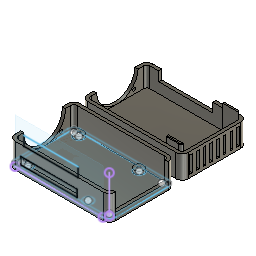
RasPi + Relay Shield (Autodesk Fusion 360 design; units mm, degrees)
Autodesk Fusion 360 part; units mm, degrees
sketch "Sketch1" plane through (0, 0, 0) normal (0, 0, 1) x (1, 0, 0)
  line L0 (-22.9024, 22.7432) -> (61.5976, 22.7432)
  line L1 (64.5976, 19.7432) -> (64.5976, -30.7568)
  line L2 (61.5976, -33.7568) -> (-22.9024, -33.7568)
  line L3 (-25.9024, -30.7568) -> (-25.9024, 19.7432)
  arc A0 (-22.9024, 22.7432) -> (-25.9024, 19.7432) centre (-22.9024, 19.7432) ccw
  arc A1 (-25.9024, -30.7568) -> (-22.9024, -33.7568) centre (-22.9024, -30.7568) ccw
  arc A2 (61.5976, -33.7568) -> (64.5976, -30.7568) centre (61.5976, -30.7568) ccw
  arc A3 (64.5976, 19.7432) -> (61.5976, 22.7432) centre (61.5976, 19.7432) ccw
  circle A4 centre (-17.4024, -30.0068) radius 1.625
  circle A5 centre (40.5976, -30.0068) radius 1.625
  circle A6 centre (40.5976, 18.9932) radius 1.625
  circle A7 centre (-17.4024, 18.9932) radius 1.625
  arc A8 (-22.9024, 25.7432) -> (-28.9024, 19.7432) centre (-22.9024, 19.7432) ccw
  line L4 (-28.9024, -30.7568) -> (-28.9024, 19.7432)
  arc A9 (-28.9024, -30.7568) -> (-22.9024, -36.7568) centre (-22.9024, -30.7568) ccw
  line L5 (61.5976, -36.7568) -> (-22.9024, -36.7568)
  arc A10 (61.5976, -36.7568) -> (67.5976, -30.7568) centre (61.5976, -30.7568) ccw
  line L6 (67.5976, 19.7432) -> (67.5976, -30.7568)
  arc A11 (67.5976, 19.7432) -> (61.5976, 25.7432) centre (61.5976, 19.7432) ccw
  line L7 (-22.9024, 25.7432) -> (61.5976, 25.7432)
  circle A12 centre (-17.4024, 18.9932) radius 4.5
  circle A13 centre (40.5976, 18.9932) radius 4.5
  circle A14 centre (-17.4024, -30.0068) radius 4.5
  circle A15 centre (40.5976, -30.0068) radius 4.5
  line L8 (64.5976, -30.7568) -> (67.5976, -30.7568)
  line L9 (64.5976, 19.7432) -> (67.5976, 19.7432)
  line L10 (-28.9024, 14.4932) -> (-25.9024, 14.4932)
  line L11 (-28.9024, -25.5068) -> (-25.9024, -25.5068)
  point P0 (-25.9024, 22.7432)
  point P1 (64.5976, 22.7432)
  point P2 (-25.9024, -33.7568)
  dimension "d1" = 90.5
  dimension "d2" = 56.5
  dimension "d3" = 3
  dimension "d4" = 3
  dimension "d5" = 3
  dimension "d6" = 3
  dimension "d8" = 3.25
  dimension "d9" = 3.25
  dimension "d10" = 3.25
  dimension "d12" = 58
  dimension "d14" = 3.25
  dimension "d15" = 3.75
  dimension "d18" = 49
  dimension "d20" = 3.75
  dimension "d21" = 58
  dimension "d22" = 3
  dimension "d23" = 49
  dimension "d24" = 9
  dimension "d25" = 9
  dimension "d26" = 9
  dimension "d27" = 9
  dimension "d28" = 40
  dimension "d29" = 11.25
  dimension "d65" = 24
  constraint perpendicular L0 L1
  constraint parallel L0 L2
  constraint parallel L1 L3
  constraint horizontal L0
  constraint coincident P0 L0
  constraint coincident P0 L3
  constraint tangent L0 A0
  constraint tangent L3 A0
  constraint coincident P2 L3
  constraint coincident P2 L2
  constraint tangent L3 A1
  constraint tangent L2 A1
  constraint tangent L2 A2
  constraint tangent L1 A2
  constraint coincident P1 L0
  constraint coincident P1 L1
  constraint tangent L0 A3
  constraint tangent L1 A3
  constraint concentric A7 A12
  constraint concentric A6 A13
  constraint concentric A4 A14
  constraint concentric A5 A15
  constraint perpendicular L1 L8
  constraint perpendicular L6 L9
  constraint coincident L4 L10.start
  constraint coincident L3 L10.end
  constraint perpendicular L3 L10
  constraint coincident L4 L11.start
  constraint coincident L3 L11.end
  constraint perpendicular L3 L11
  measures "d1" distance of P0 P1
  measures "d2" distance of P0 P2
  measures "d3" radius of A0
  measures "d4" radius of A1
  measures "d5" radius of A2
  measures "d6" radius of A3
  measures "d8" diameter of A4
  measures "d9" diameter of A5
  measures "d10" diameter of A6
  measures "d12" horizontal distance of A4.centre A5.centre
  measures "d14" diameter of A7
  measures "d15" distance of L0 A7.centre
  measures "d18" distance of A4.centre A7.centre
  measures "d20" distance of L0 A6.centre
  measures "d21" distance of A6.centre A7.centre
  measures "d22" distance of A0
  measures "d23" distance of A5.centre A6.centre
  measures "d24" diameter of A12
  measures "d25" diameter of A13
  measures "d26" diameter of A14
  measures "d27" diameter of A15
  measures "d28" distance of L10 L11
  measures "d29" distance of L5 L11
  measures "d65" distance of L1 A6.centre
extrude "Extrude1" add sketch "Sketch1" against normal blind 3 makes body 1
extrude "Extrude2" add sketch "Sketch1" along normal blind 3 contours L0 A12 | L0 A12 | L0 A13 | L0 A13 | L2 A14 | L2 A14 | L2 A15 | L2 A15 bodies 1
extrude "Extrude3" add sketch "Sketch1" along normal blind 4 contours L1 L6 L8 L9 bodies 1
extrude "Extrude4" add sketch "Sketch1" along normal blind 40 contours L0 L3 A0 A3 A8 L4 A11 L7 A12 A13 L9 L10 | L0 A12 | L0 A13 | L2 L3 A1 A2 L4 A9 L5 A10 A14 A15 L8 L11 | L2 A14 | L2 A15 picked at (-17.1836, 22.9772) picked at (41.0077, 23.0848) picked at (-16.7645, -33.8643) picked at (41.2355, -33.8643) bodies 1
sketch "Sketch2" plane through (-28.9024, 0, 0) normal (-1, 0, 0) x (0, -1, 0)
  line L0 (25.5068, 0) -> (-14.4932, 0)
  line L1 (-14.4932, 0) -> (-14.4932, 40)
  line L2 (-14.4932, 40) -> (-19.7432, 40)
  line L3 (-19.7432, 40) -> (-19.7432, -3)
  line L4 (-19.7432, -3) -> (30.7568, -3)
  line L5 (30.7568, -3) -> (30.7568, 40)
  line L6 (30.7568, 40) -> (25.5068, 40)
  line L7 (25.5068, 40) -> (25.5068, 0)
  circle A0 centre (5.5068, 20) radius 20
  line L8 (30.7568, 0) -> (-19.7432, 0)
  line L9 (-14.4932, 40) -> (25.5068, 40)
  circle A1 centre (-10.4932, 36) radius 1.45
  circle A2 centre (21.5068, 36) radius 1.45
  circle A3 centre (-10.4932, 4) radius 1.45
  circle A4 centre (21.5068, 4) radius 1.45
  dimension "d38" = 40
  dimension "d39" = 20
  dimension "d40" = 20
  dimension "d41" = 2.9
  dimension "d42" = 4
  dimension "d43" = 4
  dimension "d46" = 32
  dimension "d47" = -32
  constraint coincident L1.end L2.start
  constraint coincident L6.end L7.start
  measures "d38" diameter of A0
  measures "d39" distance of L7 A0.centre
  measures "d40" distance of A0.centre L8
  measures "d41" diameter of A1
  measures "d42" distance of L9 A1.centre
  measures "d43" distance of L1 A1.centre
extrude "Extrude5" add sketch "Sketch2" against normal blind 3 contours L0 L7 A0 L8 | L0 L1 A0 L8 | L7 A0 L9 | L1 A0 L9 bodies 1
extrude "Extrude6" add sketch "Sketch1" along normal blind 3 from surface at 40 contours L0 L3 A0 A3 A8 L4 A11 L7 A12 A13 L9 L10 | L0 L1 L2 L3 A0 A1 A2 A3 A12 A13 A14 A15 | L0 A12 | L0 A12 | L3 L4 L10 L11 | L0 A13 | L0 A13 | L2 L3 A1 A2 L4 A9 L5 A10 A14 A15 L8 L11 | L1 L6 L8 L9 | L2 A14 | L2 A14 | L2 A15 | L2 A15 | A4 | A5 | A6 | A7 bodies 1
sketch "Sketch3" plane through (0, -36.7568, 0) normal (0, -1, 0) x (1, 0, 0)
  line L0 (-22.9024, 43) -> (-22.9024, -3)
  line L1 (-22.9024, -3) -> (61.5976, -3)
  line L2 (61.5976, -3) -> (61.5976, 43)
  line L3 (61.5976, 43) -> (-22.9024, 43)
  line L4 (61.5976, 0) -> (-22.9024, 0)
  line L5 (-17.4024, 11) -> (-17.4024, 4)
  line L6 (-17.4024, 4) -> (36.5976, 4)
  line L7 (36.5976, 4) -> (36.5976, 11)
  line L8 (36.5976, 11) -> (-17.4024, 11)
  line L9 (-14.4024, 21) -> (37.5976, 21)
  line L10 (-14.4024, 21) -> (-14.4024, 30)
  line L11 (37.5976, 21) -> (37.5976, 30)
  line L12 (37.5976, 30) -> (-14.4024, 30)
  line L13 (67.5976, 4) -> (67.5976, 40)
  dimension "d56" = 7
  dimension "d57" = 54
  dimension "d58" = 4
  dimension "d59" = 21
  dimension "d60" = 52
  dimension "d62" = 9
  dimension "d68" = 30
  dimension "d69" = 31
  constraint perpendicular L5 L6
  constraint parallel L5 L7
  constraint parallel L6 L8
  constraint vertical L5
  constraint horizontal L9
  constraint perpendicular L9 L10
  constraint parallel L10 L11
  measures "d56" distance of L5.start L5.end
  measures "d57" distance of L5.start L7.end
  measures "d58" distance of L4 L6
  measures "d59" distance of L4 L9
  measures "d60" distance of L9.start L9.end
  measures "d62" distance of L9.start L10.end
  measures "d68" distance of L11 L13
  measures "d69" distance of L7 L13
extrude "Extrude7" cut sketch "Sketch3" against normal blind 3 contours L5 L6 L7 L8 | L9 L10 L11 L12 bodies 1
ref_plane "WorkPlane1" through (19.3476, -5.5068, 21) normal (0, 0, 1) x (1, 0, 0)
sketch "Sketch4" plane through (0, 0, 40) normal (0, 0, -1) x (1, 0, 0)
  line L0 (64.5976, -19.7432) -> (67.5976, -19.7432)
  line L1 (67.5976, -19.7432) -> (67.5976, 30.7568)
  line L2 (67.5976, 30.7568) -> (64.5976, 30.7568)
  arc A0 (64.5976, 30.7568) -> (61.5976, 33.7568) centre (61.5976, 30.7568) ccw
  line L3 (61.5976, 33.7568) -> (-22.9024, 33.7568)
  arc A1 (-22.9024, 33.7568) -> (-25.9024, 30.7568) centre (-22.9024, 30.7568) ccw
  line L4 (-25.9024, 30.7568) -> (-25.9024, 5.5068)
  line L5 (-25.9024, 5.5068) -> (-25.9024, -19.7432)
  arc A2 (-25.9024, -19.7432) -> (-22.9024, -22.7432) centre (-22.9024, -19.7432) ccw
  line L6 (-22.9024, -22.7432) -> (61.5976, -22.7432)
  arc A3 (61.5976, -22.7432) -> (64.5976, -19.7432) centre (61.5976, -19.7432) ccw
  line L7 (64.5976, 30.7568) -> (64.5976, -19.7432)
  constraint coincident L2.end A0.start
  constraint coincident L0.start A3.end
extrude "Extrude8" add sketch "Sketch4" along normal blind 19 contours L0 L1 L2 L7 bodies 1
sketch "Sketch5" plane through (67.5976, 0, 0) normal (1, 0, 0) x (0, 1, 0)
  line L0 (19.7432, 21) -> (19.7432, 43)
  line L1 (19.7432, 43) -> (-30.7568, 43)
  line L2 (-30.7568, 43) -> (-30.7568, 21)
  line L3 (-30.7568, 21) -> (19.7432, 21)
  line L4 (-29.2586, 40) -> (-29.2586, 24)
  line L5 (-29.2586, 24) -> (-26.7586, 24)
  line L6 (-26.7586, 24) -> (-26.7586, 40)
  line L7 (-26.7586, 40) -> (-29.2586, 40)
  line L8 (-30.7568, 40) -> (-5.5068, 40)
  line L9 (-20.33, 24) -> (-20.33, 40)
  line L10 (-20.33, 40) -> (-22.83, 40)
  line L11 (-22.83, 40) -> (-22.83, 24)
  line L12 (-22.83, 24) -> (-20.33, 24)
  line L13 (-13.9015, 24) -> (-13.9015, 40)
  line L14 (-13.9015, 40) -> (-16.4015, 40)
  line L15 (-16.4015, 40) -> (-16.4015, 24)
  line L16 (-16.4015, 24) -> (-13.9015, 24)
  line L17 (-7.4729, 24) -> (-7.4729, 40)
  line L18 (-7.4729, 40) -> (-9.9729, 40)
  line L19 (-9.9729, 40) -> (-9.9729, 24)
  line L20 (-9.9729, 24) -> (-7.4729, 24)
  line L21 (-1.0443, 24) -> (-1.0443, 40)
  line L22 (-1.0443, 40) -> (-3.5443, 40)
  line L23 (-3.5443, 40) -> (-3.5443, 24)
  line L24 (-3.5443, 24) -> (-1.0443, 24)
  line L25 (5.3842, 24) -> (5.3842, 40)
  line L26 (5.3842, 40) -> (2.8842, 40)
  line L27 (2.8842, 40) -> (2.8842, 24)
  line L28 (2.8842, 24) -> (5.3842, 24)
  line L29 (11.8128, 24) -> (11.8128, 40)
  line L30 (11.8128, 40) -> (9.3128, 40)
  line L31 (9.3128, 40) -> (9.3128, 24)
  line L32 (9.3128, 24) -> (11.8128, 24)
  line L33 (18.2414, 24) -> (18.2414, 40)
  line L34 (18.2414, 40) -> (15.7414, 40)
  line L35 (15.7414, 40) -> (15.7414, 24)
  line L36 (15.7414, 24) -> (18.2414, 24)
  dimension "d73" = 2.5
  dimension "d76" = 45
  dimension "d77" = 0
  constraint perpendicular L4 L5
  constraint parallel L4 L6
  constraint parallel L5 L7
  constraint perpendicular L4 L8
  constraint coincident L4.start L8
  measures "d73" distance of L4.start L6.end
extrude "Extrude9" cut sketch "Sketch5" against normal up to surface (3 mm away) contours L4 L5 L6 L7 L8 | L8 L9 L10 L11 L12 | L8 L13 L14 L15 L16 | L8 L17 L18 L19 L20 | L21 L22 L23 L24 | L25 L26 L27 L28 | L29 L30 L31 L32 | L33 L34 L35 L36 bodies 1
split "Split2" by plane through (19.3476, -5.5068, 21) normal (0, 0, 1) bodies 1 makes body 2 at (33.4309, -15.9234, 43)
move_body "Move1" bodies 2 to x (1, 0, 0) y (0, -1, 0) z (0, 0, -1) at (0, 58.9865, 40)
sketch "Sketch6" plane through (0, 0, 0) normal (0, 0, 1) x (-1, 0, 0)
  line L0 (-64.5976, -39.2432) -> (-64.5976, -40.7451)
  line L1 (-64.5976, -40.7451) -> (-67.5976, -40.7451)
  line L2 (-67.5976, -40.7451) -> (-67.5976, -43.2451)
  line L3 (-67.5976, -43.2451) -> (-64.5976, -43.2451)
  line L4 (-64.5976, -43.2451) -> (-64.5976, -47.1737)
  line L5 (-64.5976, -47.1737) -> (-67.5976, -47.1737)
  line L6 (-67.5976, -47.1737) -> (-67.5976, -49.6737)
  line L7 (-67.5976, -49.6737) -> (-64.5976, -49.6737)
  line L8 (-64.5976, -49.6737) -> (-64.5976, -53.6022)
  line L9 (-64.5976, -53.6022) -> (-67.5976, -53.6022)
  line L10 (-67.5976, -53.6022) -> (-67.5976, -56.1022)
  line L11 (-67.5976, -56.1022) -> (-64.5976, -56.1022)
  line L12 (-64.5976, -56.1022) -> (-64.5976, -60.0308)
  line L13 (-64.5976, -60.0308) -> (-67.5976, -60.0308)
  line L14 (-67.5976, -60.0308) -> (-67.5976, -62.5308)
  line L15 (-67.5976, -62.5308) -> (-64.5976, -62.5308)
  line L16 (-64.5976, -62.5308) -> (-64.5976, -66.4594)
  line L17 (-64.5976, -66.4594) -> (-67.5976, -66.4594)
  line L18 (-67.5976, -66.4594) -> (-67.5976, -68.9594)
  line L19 (-67.5976, -68.9594) -> (-64.5976, -68.9594)
  line L20 (-64.5976, -68.9594) -> (-64.5976, -72.888)
  line L21 (-64.5976, -72.888) -> (-67.5976, -72.888)
  line L22 (-67.5976, -72.888) -> (-67.5976, -75.388)
  line L23 (-67.5976, -75.388) -> (-64.5976, -75.388)
  line L24 (-64.5976, -75.388) -> (-64.5976, -79.3165)
  line L25 (-64.5976, -79.3165) -> (-67.5976, -79.3165)
  line L26 (-67.5976, -79.3165) -> (-67.5976, -81.8165)
  line L27 (-67.5976, -81.8165) -> (-64.5976, -81.8165)
  line L28 (-64.5976, -81.8165) -> (-64.5976, -85.7451)
  line L29 (-64.5976, -85.7451) -> (-67.5976, -85.7451)
  line L30 (-67.5976, -85.7451) -> (-67.5976, -88.2451)
  line L31 (-67.5976, -88.2451) -> (-64.5976, -88.2451)
  line L32 (-64.5976, -88.2451) -> (-64.5976, -89.7432)
  arc A0 (-64.5976, -89.7432) -> (-61.5976, -92.7432) centre (-61.5976, -89.7432) ccw
  line L33 (-61.5976, -92.7432) -> (22.9024, -92.7432)
  arc A1 (22.9024, -92.7432) -> (25.9024, -89.7432) centre (22.9024, -89.7432) ccw
  line L34 (25.9024, -89.7432) -> (25.9024, -64.4932)
  line L35 (25.9024, -64.4932) -> (25.9024, -39.2432)
  arc A2 (25.9024, -39.2432) -> (22.9024, -36.2432) centre (22.9024, -39.2432) ccw
  line L36 (22.9024, -36.2432) -> (-61.5976, -36.2432)
  arc A3 (-61.5976, -36.2432) -> (-64.5976, -39.2432) centre (-61.5976, -39.2432) ccw
  line L37 (-49.426, -36.2432) -> (-49.426, -38.2432)
  line L38 (-49.426, -38.2432) -> (-64.426, -38.2432)
  line L39 (-49.426, -92.7432) -> (-49.426, -90.7432)
  line L40 (-49.426, -90.7432) -> (-64.426, -90.7432)
  dimension "d80" = 2
  dimension "d81" = 15
  dimension "d82" = 2
  dimension "d83" = 15
  constraint coincident L36 L37.start
  constraint coincident A3 L38.end
  constraint perpendicular L37 L38
  constraint coincident L33 L39.start
  constraint coincident A0 L40.end
  constraint perpendicular L39 L40
  measures "d80" distance of L37.start L37.end
  measures "d81" distance of L37.end L38.end
  measures "d82" distance of L39.start L39.end
  measures "d83" distance of L39.end L40.end
extrude "Extrude10" add sketch "Sketch6" along normal blind 25 contours L36 A3 L37 L38 | A0 L33 L39 L40 bodies 2
chamfer "Chamfer1" distance 0.5 angle 45 4 edges at (55.5118, 36.2432, 25) (63.3296, 36.7938, 25) (63.3296, 92.1927, 25) (55.5118, 92.7432, 25) on bodies 2
sketch "Sketch7" plane through (0, 0, -3) normal (0, 0, -1) x (1, 0, 0)
  circle A0 centre (-17.4024, 30.0068) radius 1.625
  circle A1 centre (-17.4024, -18.9932) radius 1.625
  circle A2 centre (40.5976, 30.0068) radius 1.625
  circle A3 centre (40.5976, -18.9932) radius 1.625
  arc A4 (-22.9024, 36.7568) -> (-28.9024, 30.7568) centre (-22.9024, 30.7568) ccw
  line L0 (-28.9024, 30.7568) -> (-28.9024, -19.7432)
  arc A5 (-28.9024, -19.7432) -> (-22.9024, -25.7432) centre (-22.9024, -19.7432) ccw
  line L1 (-22.9024, -25.7432) -> (61.5976, -25.7432)
  arc A6 (61.5976, -25.7432) -> (67.5976, -19.7432) centre (61.5976, -19.7432) ccw
  line L2 (67.5976, -19.7432) -> (67.5976, 30.7568)
  arc A7 (67.5976, 30.7568) -> (61.5976, 36.7568) centre (61.5976, 30.7568) ccw
  line L3 (61.5976, 36.7568) -> (-22.9024, 36.7568)
  circle A8 centre (-17.4024, 30.0068) radius 2.75
  circle A9 centre (40.5976, 30.0068) radius 2.75
  circle A10 centre (-17.4024, -18.9932) radius 2.75
  circle A11 centre (40.5976, -18.9932) radius 2.75
  dimension "d87" = 5.5
  dimension "d88" = 5.5
  dimension "d89" = 5.5
  dimension "d90" = 5.5
  constraint concentric A0 A8
  constraint concentric A2 A9
  constraint concentric A1 A10
  constraint concentric A3 A11
  measures "d87" diameter of A8
  measures "d88" diameter of A9
  measures "d89" diameter of A10
  measures "d90" diameter of A11
extrude "Extrude11" cut sketch "Sketch7" against normal blind 2.75 contours A8 | A9 | A10 | A11 bodies 1
equation "d1 = 85.5 mm + 5 mm"
equation "d29 = ( ( 56.5 / 2 ) * 1 mm ) - 20 mm + 3 mm"
equation "d71 = 22 mm - 3 mm"
named bodies: "Bottom", "Top"
